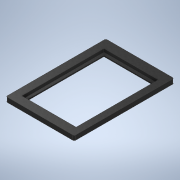
# Autodesk Inventor part: plate-holder
Saved by Autodesk Inventor 2020 (Build 240168000, 168)
## iProperties
Created: 2020-08-25
Part Number: plate-holder
Material: 常规
Document SubType Name: Sheet Metal
Designer: Dell
Density: 1 g/cm^3
Sheet Metal Rule: 默认_mm
Appearance: 菱形板 - 深灰色
Author: Dell
Autodesk Inventor part; units mm, degrees
ref_plane "YZ Plane" through (0, 0, 0) normal (1, 0, 0) x (0, 1, 0)
ref_plane "XZ Plane" through (0, 0, 0) normal (0, 1, 0) x (-1, 0, 0)
ref_plane "XY Plane" through (0, 0, 0) normal (0, 0, 1) x (1, 0, 0)
sketch "草图1" plane through (0, 0, 0) normal (0, 1, 0) x (-1, 0, 0)
  line L0 (0, 0) -> (0, -158)
  line L1 (0, -158) -> (-108, -158)
  line L2 (-108, -158) -> (-108, 0)
  line L3 (-108, 0) -> (0, 0)
  line L4 (-54.65, -78.4) -> (-11.65, -78.4)
  line L5 (-11.65, -78.4) -> (-11.65, -143.4)
  line L6 (-11.65, -143.4) -> (-97.65, -143.4)
  line L7 (-97.65, -143.4) -> (-97.65, -13.4)
  line L8 (-97.65, -13.4) -> (-11.65, -13.4)
  line L9 (-11.65, -13.4) -> (-11.65, -78.4)
  dimension "d0" = 158
  dimension "d1" = 108
  dimension "d2" = 43
  dimension "d4" = 65
  dimension "d5" = 86
  dimension "d6" = 130
  constraints: 20 end point, 7 perpendicular, 2 vertical, 1 horizontal, 1 point on line
  measures "d0" distance of L0.start L0.end
  measures "d1" distance of L0.end L1.end
  measures "d2" distance of L4.start L4.end
  measures "d4" distance of L4.end L5.end
  measures "d5" distance of L5.end L6.end
  measures "d6" distance of L6.end L7.end
extrude "拉伸1" add sketch "草图1" along normal blind 7.2
fillet "圆角1" radius 2 4 edges at (108, 3.6, 0) (108, 3.6, -158) (0, 3.6, 0) (0, 3.6, -158)
sketch "草图2" plane through (0, 0, 0) normal (0, -1, 0) x (1, 0, 0)
  line L0 (11.65, -143.4) -> (97.65, -143.4) projected
  line L1 (11.65, -143.4) -> (11.65, -139.4)
  line L2 (11.65, -13.4) -> (11.65, -143.4) projected
  line L3 (11.65, -139.4) -> (15.65, -139.4)
  line L4 (15.65, -139.4) -> (93.65, -139.4)
  line L5 (93.65, -139.4) -> (93.65, -17.4)
  line L6 (93.65, -17.4) -> (15.65, -17.4)
  line L7 (15.65, -17.4) -> (15.65, -139.4)
  line L8 (97.65, -13.4) -> (11.65, -13.4) projected
  line L9 (11.65, -143.4) -> (97.65, -143.4)
  line L10 (97.65, -143.4) -> (97.65, -13.4)
  line L11 (97.65, -13.4) -> (11.65, -13.4)
  line L12 (11.65, -13.4) -> (11.65, -143.4)
  point P0 (0, 0)
  point P1 (97.65, -143.4)
  dimension "d10" = 4
  dimension "d11" = 4
  dimension "d12" = 78
  dimension "d13" = 122
  constraints: 20 end point, 4 parallel, 3 perpendicular, 2 horizontal, 1 point on line
  measures "d10" distance of L0.start L1.end
  measures "d11" distance of L1.end L3.end
  measures "d12" distance of L6.end L5.end
  measures "d13" distance of L5.end L4.end
extrude "拉伸2" add sketch "草图2" against normal blind 2
equation "\"折弯半径\" = 厚度"
equation "\"折弯释压宽度\" = 厚度"
equation "\"折弯释压深度\" = 0.5 * 厚度"
equation "\"拐角释压尺寸\" = 4 * 厚度"
equation "\"最小余量\" = 2 * 厚度"
equation "\"过渡半径\" = 折弯半径"
equation "\"Jacobi半径尺寸\" = 折弯半径"
equation "\"间隙大小\" = 厚度"
equation "\"厚度\" = 0.5"
